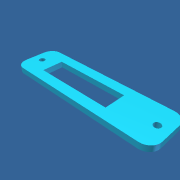
# Autodesk Inventor part: Acrylic_YawServoSupport_3
Saved by Autodesk Inventor 2012 (Build 160160000, 160)
## iProperties
Created: 2014-03-29
Part Number: Acrylic_YawServoSupport_3
Material: Default
Document SubType Name: Modeling
Designer: Admin
Density: 1 g/cm^3
Author: Admin
Autodesk Inventor part; units mm, degrees
ref_plane "YZ Plane" through (0, 0, 0) normal (1, 0, 0) x (0, 1, 0)
ref_plane "XZ Plane" through (0, 0, 0) normal (0, 1, 0) x (-1, 0, 0)
ref_plane "XY Plane" through (0, 0, 0) normal (0, 0, 1) x (1, 0, 0)
sketch "Sketch1" plane through (0, 0, 0) normal (0, 0, 1) x (1, 0, 0)
  line L0 (-30, 10) -> (30, 10)
  line L1 (35, 5) -> (35, -5)
  line L2 (30, -10) -> (-30, -10)
  line L3 (-35, -5) -> (-35, 5)
  line L4 (-50.4497, 0) -> (50.4497, 0) projected
  line L5 (0, -15.4497) -> (0, 15.4497) projected
  arc A0 (-30, 10) -> (-35, 5) centre (-30, 5) ccw
  arc A1 (-35, -5) -> (-30, -10) centre (-30, -5) ccw
  arc A2 (30, -10) -> (35, -5) centre (30, -5) ccw
  arc A3 (35, 5) -> (30, 10) centre (30, 5) ccw
  line L6 (-22.5, 5) -> (12.5, 5)
  line L7 (12.5, 5) -> (12.5, -5)
  line L8 (12.5, -5) -> (-22.5, -5)
  line L9 (-22.5, -5) -> (-22.5, 5)
  circle A4 centre (-30, 0) radius 1.5
  circle A5 centre (30, 0) radius 1.5
  point P0 (0, 0)
  point P1 (-35, 10)
  point P2 (35, -10)
  point P3 (35, 10)
  point P4 (-35, -10)
  dimension "d2" = 70
  dimension "d3" = 35
  dimension "d4" = 20
  dimension "d5" = 10
  dimension "d6" = 5
  dimension "d7" = 35
  dimension "d8" = 12.5
  dimension "d9" = 3
  dimension "d10" = 3
  constraints: 16 end point, 10 point on line, 8 point on circle, 8 tangent, 6 centre point, 4 parallel, 3 equal radius, 2 horizontal, 2 perpendicular
  measures "d2" distance of point (-35, 10) point (35, 10)
  measures "d3" distance between parallel lines of L1 L5
  measures "d4" distance of point (35, 10) point (35, -10)
  measures "d5" distance between parallel lines of L4 L0
  measures "d6" radius of A0
  measures "d7" distance of L7.end L8.end
  measures "d8" distance between parallel lines of L3 L9
  measures "d9" diameter of A4
  measures "d10" diameter of A5
extrude "Extrusion1" add sketch "Sketch1" along normal blind 2.8 contours L0 L5 L6 L9 L4 A4 L3 A0 | L0 A3 L1 L4 A5 L7 L6 L5 | L4 A4 L9 L8 L5 L2 A1 L3 | L1 A2 L2 L5 L8 L7 L4 A5
equation "\"d3\" = 0.5 * d2"
equation "\"d5\" = 0.5 * d4"
body "Solid1"
